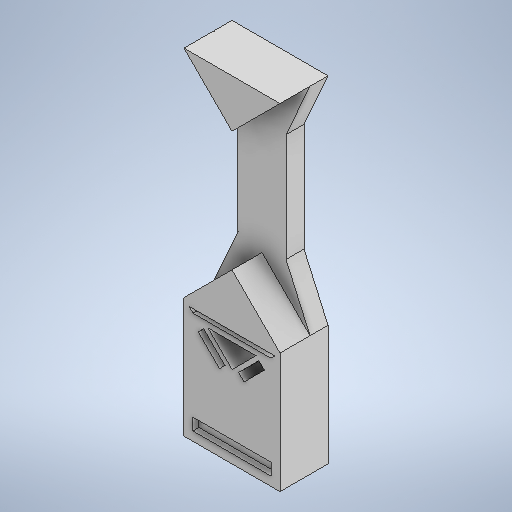
# Autodesk Inventor part: Connecting pt.2
Saved by Autodesk Inventor 2025.2 (Build 292293000, 293)
## iProperties
Created: 2025-04-14
Part Number: Connecting pt.2
Material: Generic
Document SubType Name: Modeling
Designer: 1khanhan2
Density: 1 g/cm^3
Appearance: Default
Author: 1khanhan2
Autodesk Inventor part; units mm, degrees
ref_plane "YZ Plane" through (0, 0, 0) normal (1, 0, 0) x (0, 1, 0)
ref_plane "XZ Plane" through (0, 0, 0) normal (0, 1, 0) x (-1, 0, 0)
ref_plane "XY Plane" through (0, 0, 0) normal (0, 0, 1) x (1, 0, 0)
sketch "Sketch1" plane through (0, 0, 0) normal (0, 0, 1) x (1, 0, 0)
  line L0 (0, 0) -> (0, 20)
  line L1 (0, 20) -> (16, 20)
  line L2 (16, 20) -> (16, 0)
  line L3 (16, 0) -> (0, 0)
  line L4 (8, 28) -> (0, 20)
  line L5 (8, 28) -> (16, 20)
  line L6 (0, 0) -> (0, 5)
  line L7 (0, 0) -> (0, 1.5)
  line L8 (0, 5) -> (0, 3.5)
  line L9 (1.5, 3.5) -> (1.5, 1.5)
  line L10 (1.5, 3.5) -> (14.5, 3.5)
  line L11 (14.5, 3.5) -> (14.5, 1.5)
  line L12 (14.5, 1.5) -> (1.5, 1.5)
  line L13 (14.5, 18.5) -> (15.1649, 19.1649)
  line L14 (15.1649, 19.1649) -> (0.8351, 19.1649)
  line L15 (0.8351, 19.1649) -> (1.5, 18.5)
  line L16 (1.5, 18.5) -> (14.5, 18.5)
  line L17 (12, 17.6183) -> (4, 17.6183)
  line L18 (4, 17.6183) -> (8.0319, 13.6184)
  line L19 (8.0319, 13.6184) -> (12, 17.6183)
  line L20 (12.4747, 17.1474) -> (13.3985, 16.231)
  line L21 (13.3985, 16.231) -> (10.016, 12.8213)
  line L22 (10.016, 12.8213) -> (9.0922, 13.7377)
  line L23 (9.0922, 13.7377) -> (12.4747, 17.1474)
  line L24 (6.8378, 13.6184) -> (3.2805, 17.1474)
  line L25 (3.2805, 17.1474) -> (2.3714, 16.231)
  line L26 (2.3714, 16.231) -> (5.9286, 12.702)
  line L27 (5.9286, 12.702) -> (6.8378, 13.6184)
  dimension "d0" = 20
  dimension "d1" = 16
  dimension "d3" = 5
  dimension "d7" = 1.5
  dimension "d9" = 13
  constraints: 56 end point, 14 perpendicular, 4 point on line, 2 horizontal, 1 parallel, 1 vertical
  measures "d0" distance of L0.start L0.end
  measures "d1" distance of L0.end L1.end
  measures "d3" distance of L0.start L6.end
  measures "d7" distance of L7.end L9.end
  measures "d9" distance of L9.start L10.end
extrude "Extrusion1" add sketch "Sketch1" along normal blind 5
extrude "Extrusion2" add sketch "Sketch1" along normal blind 4 contours L10 L11 L12 L9
sketch "Sketch2" plane through (0, 0, 0) normal (0, 0, -1) x (-1, 0, 0)
  line L0 (-16, 20) -> (-8, 28) projected
  line L1 (-16, 20) -> (0, 20)
  line L2 (0, 20) -> (-8, 28)
  line L3 (-16, 20) -> (-16, 56)
  line L4 (-16, 20) -> (20, 20) construction
  line L5 (-16, 56) -> (0, 56)
  line L6 (0, 56) -> (0, 20)
  line L7 (-16, 56) -> (-8, 48)
  line L8 (-16, 56) -> (-4.6863, 56) construction
  line L9 (-8, 48) -> (0, 56)
  point P0 (0, 0)
  dimension "d12" = 36
  dimension "d13" = 90
  dimension "d14" = 45
  constraints: 18 end point, 4 perpendicular, 3 horizontal, 2 equal length, 1 vertical
  measures "d12" distance of L0.start L3.end
  measures "d13" angle of L4 L3
  measures "d14" angle of L7 L8
extrude "Extrusion3" add sketch "Sketch2" against normal blind 5 contours L5 L9 L7
sketch "Sketch3" plane through (0, 0, 0) normal (0, 0, -1) x (-1, 0, 0)
  line L0 (0, 56) -> (-8, 48) projected
  line L1 (-16, 0) -> (-16, 20) projected
  line L2 (0, 56) -> (-16, 56)
  line L3 (-16, 56) -> (-16, 0)
  line L4 (-16, 0) -> (0, 0)
  line L5 (0, 0) -> (0, 56)
  line L6 (-16, 20) -> (-8, 28) projected
  line L7 (-16, 20) -> (0, 20)
  line L8 (-8, 28) -> (0, 20) projected
  line L9 (-8, 28) -> (-8, 48)
  line L10 (-16, 56) -> (-8, 38)
  line L11 (0, 56) -> (-8, 38)
  line L12 (-8, 38) -> (0, 20)
  line L13 (-8, 38) -> (-16, 20)
  line L14 (-12, 47) -> (-12, 29)
  line L15 (-4, 47) -> (-4, 29)
  point P0 (0, 0)
  constraints: 24 end point, 5 midpoint, 3 equal length, 3 perpendicular, 1 horizontal, 1 point on line
extrude "Extrusion4" add sketch "Sketch3" along normal blind 3 contours L11 L9 L0 | L0 L9 L10 L2 | L5 L4 L1 L7 | L7 L6 L8 | L8 L9 L12 | L15 L12 L11 | L13 L14 L10 | L9 L6 L13
body "Solid1"
